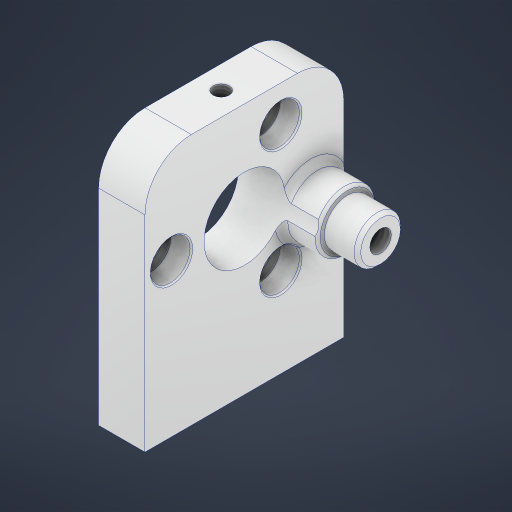
# Autodesk Inventor part: Lagerblock
Saved by Autodesk Inventor 2024.1 (Build 281209000, 209)
## iProperties
Created: 2023-10-17
Part Number: Lagerblock
Material: Aluminium 6061
Document SubType Name: Modeling
Designer: Fabian
Density: 2.7 g/cm^3
Appearance: Aluminium - flach
Author: Fabian
Autodesk Inventor part; units mm, degrees
ref_plane "YZ Plane" through (0, 0, 0) normal (1, 0, 0) x (0, 1, 0)
ref_plane "XZ Plane" through (0, 0, 0) normal (0, 1, 0) x (-1, 0, 0)
ref_plane "XY Plane" through (0, 0, 0) normal (0, 0, 1) x (1, 0, 0)
sketch "Skizze1" plane through (0, 0, 0) normal (1, 0, 0) x (0, 1, 0)
  line L0 (-20, 15) -> (13, 15)
  line L1 (20, 8) -> (20, -8)
  line L2 (13, -15) -> (-20, -15)
  line L3 (-20, -15) -> (-20, 15)
  line L4 (-20, 15) -> (20, -15) construction
  line L5 (20, 15) -> (-20, -15) construction
  circle A0 centre (5, 0) radius 6.1
  circle A1 centre (5, 11) radius 1.6
  circle A2 centre (5, 11) radius 1.6
  circle A3 centre (-4.5263, -5.5) radius 1.6
  circle A4 centre (-4.5263, -5.5) radius 1.6
  circle A5 centre (14.5263, -5.5) radius 1.6
  circle A6 centre (14.5263, -5.5) radius 1.6
  circle A7 centre (5, 0) radius 10.4
  arc A8 (20, 8) -> (13, 15) centre (13, 8) ccw
  arc A9 (13, -15) -> (20, -8) centre (13, -8) ccw
  line L6 (5, 6.2) -> (5, -6.2)
  line L7 (5, 0) -> (2.3083, -10.0456)
  circle A10 centre (2.3083, -10.0456) radius 4.5
  circle A11 centre (2.3083, -10.0456) radius 3.5
  line L8 (-20, 0) -> (-18, 0)
  line L9 (-18, 0) -> (-18, -15)
  line L10 (-18, 0) -> (-18, 15)
  point P0 (0, 0)
  point P1 (31.9658, 28.1951)
  point P2 (7.3809, -10.1238)
  point P3 (4.4211, -6.0725)
  point P4 (2.4651, -5.5484)
  dimension "d0" = 40
  dimension "d1" = 30
  dimension "d2" = 20.8
  dimension "d5" = 7
  dimension "d46" = 10.4
  dimension "d47" = 15
  dimension "d48" = 9
  dimension "d49" = 7
  dimension "d60" = 2
  dimension "d71" = 12.2
  constraints: 22 end point, 12 centre point, 7 point on line, 6 coincident, 4 point on circle, 4 tangent, 3 midpoint, 2 horizontal, 2 parallel, 2 perpendicular, 1 equal radius, 1 vertical
  measures "d0" distance of L4.end L2.end
  measures "d1" distance of L5.start L4.end
  measures "d2" diameter of A7
  measures "d5" radius of A8
  measures "d46" distance of L7.start L7.end
  measures "d47" angle of L6 L7
  measures "d48" diameter of A10
  measures "d49" diameter of A11
  measures "d60" distance of L8.start L8.end
  measures "d71" diameter of A0
extrude "Extrusion1" add sketch "Skizze1" against normal blind 7 contours L0 A8 L1 A9 L2 L9 L10 | A0 A10 A7 A3 A1 A5 | A0 L7 A11 A7 A10 | A10 A7 A11 L7 A0 | A7 A11 A10 | A11 A7 L7 | L7 A7 A11 | A7 A3 | A3 A7 | A7 A11 | A7 A5 | A5 A7 | A7 A1 | A1 A7
extrude "Extrusion2" add sketch "Skizze1" along normal blind 10.5 and the other way blind 5 contours A11 A7 L7 | L7 A7 A11 | A7 A11
chamfer "Fasen1" distance 0.5 angle 45 1 edges at (10.5, -1.1917, -10.0456)
hole "Bohrung2" at (0, 5, 11) at (0, -4.5263, -5.5) at (0, 14.5263, -5.5) direction (-1, 0, 0) diameter 3 depth 8 tip angle 118 counterbore diameter 6 counterbore depth 3.1
extrude "Extrusion4" add sketch "Skizze1" along normal blind 5.5 contours A0 L7 A11 A7 A10 | A10 A7 A11 L7 A0 | A7 A11 A10
sketch "Skizze4" plane through (10.5, 0, 0) normal (1, 0, 0) x (0, 0, -1)
  arc A0 (10.0456, 5.3083) -> (10.0456, 5.3083) centre (10.0456, 2.3083) ccw projected
  point P0 (0, 0)
  constraints: 1 coincident
hole "Bohrung4" at (10.5, 2.3083, -10.0456) direction (-1, 0, 0) diameter 3.242 depth 17.5 thread size "M4x0.7" class "6H" standard "ISO Metric profile"
fillet "Rundung2" radius 1 1 edges at (0, 1.1436, -14.3923)
sketch "Skizze5" plane through (0, -18, -15) normal (0, -1, 0) x (1, 0, 0)
  point P0 (-3.5, 22.5)
  point P1 (-3.5, 15)
  point P2 (-3.5, 7.5)
hole "Bohrung5" at (-3.5, -18, 7.5) at (-3.5, -18, 0) at (-3.5, -18, -7.5) direction (0, 1, 0) diameter 2.459 depth 8.8 tip angle 118 thread size "M3x0.5" class "6H" standard "ISO Metric profile"
chamfer "Fasen2" distance 0.2 angle 45 5 edges at (0, 5, 14) (0, 14.5263, -2.5) (0, -3.6029, -8.3544) (0, -6.3916, -3.1504) (0.0435, -2.0283, -7.1614)
sketch "Skizze8" plane through (0, 20, 8) normal (0, 1, 0) x (1, 0, 0)
  line L0 (0, 16) -> (-7, 16) projected
  line L1 (-3.5, 16) -> (-3.5, 0)
  line L2 (0, 0) -> (-7, 0) projected
  point P0 (-3.5, 8)
  constraints: 3 midpoint, 2 end point
hole "Bohrung6" at (-3.5, 20, 0) direction (0, -1, 0) diameter 2.459 depth 6 tip angle 118 thread size "M3x0.5" class "6H" standard "ISO Metric profile"
chamfer "Fasen3" distance 0.4 angle 45 1 edges at (5.5, 1.1436, -14.3923)
